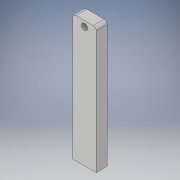
# Autodesk Inventor part: backside arm
Saved by Autodesk Inventor 2019 (Build 230136000, 136)
## iProperties
Created: 2019-10-24
Part Number: backside arm
Material: Generic
Document SubType Name: Modeling
Designer: robgr
Density: 1 g/cm^3
Appearance: Default
Author: robgr
Autodesk Inventor part; units mm, degrees
ref_plane "YZ Plane" through (0, 0, 0) normal (1, 0, 0) x (0, 1, 0)
ref_plane "XZ Plane" through (0, 0, 0) normal (0, 1, 0) x (-1, 0, 0)
ref_plane "XY Plane" through (0, 0, 0) normal (0, 0, 1) x (1, 0, 0)
sketch "Sketch1" plane through (0, 0, 0) normal (0, 0, 1) x (1, 0, 0)
  circle A0 centre (0, 0) radius 2
  line L0 (-5.5, 3.5) -> (5.5, 3.5)
  line L1 (7.5, 1.5) -> (7.5, -3.5)
  line L2 (7.5, -3.5) -> (-7.5, -3.5)
  line L3 (-7.5, -3.5) -> (-7.5, 1.5)
  arc A1 (-5.5, 3.5) -> (-7.5, 1.5) centre (-5.5, 1.5) ccw
  arc A2 (7.5, 1.5) -> (5.5, 3.5) centre (5.5, 1.5) ccw
  point P0 (7.5, 3.5)
  dimension "d0" = 4
  dimension "d1" = 15
  dimension "d2" = 7
  dimension "d3" = 7.5
  dimension "d4" = 3.5
  dimension "d5" = 2
  constraints: 8 end point, 4 point on circle, 4 tangent, 3 centre point, 2 parallel, 2 point on line, 1 coincident, 1 equal radius, 1 horizontal, 1 perpendicular
  measures "d0" diameter of A0
  measures "d1" distance of L1.end L2.end
  measures "d2" distance of point (7.5, 3.5) L1.end
  measures "d3" distance from line of L3 point (0, 0)
  measures "d4" distance from line of L2 point (0, 0)
  measures "d5" radius of A1
extrude "Extrusion1" add sketch "Sketch1" along normal blind 7
sketch "Sketch2" plane through (-7.5, -3.5, 0) normal (0, -1, 0) x (1, 0, 0)
  line L0 (15, 0) -> (13, 0) projected
  line L1 (0, 7) -> (15, 7)
  line L2 (15, 7) -> (15, 0)
  line L3 (15, 0) -> (0, 0)
  line L4 (0, 0) -> (0, 7)
  line L5 (0, 7) -> (15, 7) projected
  line L6 (0, 0) -> (0, 7) projected
  point P0 (7.5, 0)
  dimension "d8" = 0
  dimension "d9" = 0
  constraints: 8 end point, 2 parallel, 1 horizontal, 1 perpendicular
  measures "d8" distance between parallel lines of L5 L1
  measures "d9" distance between parallel lines of L6 L4
extrude "Extrusion2" add sketch "Sketch2" along normal blind 73.5
body "Solid1"
